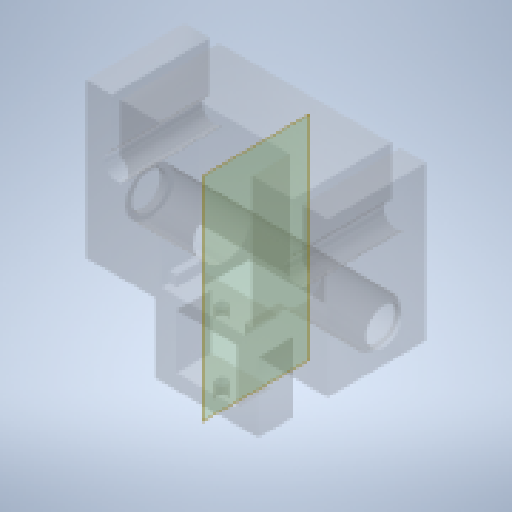
# Autodesk Inventor part: GantryHolder
Saved by Autodesk Inventor 2023 (Build 270158000, 158)
## iProperties
Created: 2022-08-28
Part Number: GantryHolder
Material: PET Plastic
Document SubType Name: Modeling
Designer: Nathann
Density: 1.541 g/cm^3
Appearance: Polycarbonate - Clear
Mass: 118.586 g
Surface Area: 221.873 cm^2
Volume: 76.9541 cm^3
Author: Nathann
Autodesk Inventor part; units mm, degrees
ref_plane "YZ Plane" through (0, 0, 0) normal (1, 0, 0) x (0, 1, 0)
ref_plane "XZ Plane" through (0, 0, 0) normal (0, 1, 0) x (-1, 0, 0)
ref_plane "XY Plane" through (0, 0, 0) normal (0, 0, 1) x (1, 0, 0)
sketch "Sketch1" plane through (0, 0, 0) normal (0, 1, 0) x (-1, 0, 0)
  arc A0 (8.5, 13.7081) -> (11.5, 13.7081) centre (10, 10) ccw
  line L0 (8.5, 20) -> (8.5, 13.7081)
  line L1 (11.5, 20) -> (11.5, 13.7081)
  line L2 (10, 20) -> (10, 18.7339)
  line L3 (20, 20) -> (10, 20)
  line L4 (8.5, 20) -> (0, 20)
  line L5 (0, 20) -> (0, 0)
  line L6 (0, 0) -> (20, 0)
  line L7 (20, 0) -> (20, 20)
  arc A1 (68.5, 13.7081) -> (71.5, 13.7081) centre (70, 10) ccw
  line L8 (68.5, 20) -> (68.5, 13.7081)
  line L9 (71.5, 20) -> (71.5, 13.7081)
  line L10 (70, 20) -> (70, 18.3732)
  line L11 (80, 20) -> (70, 20)
  line L12 (68.5, 20) -> (60.9559, 20)
  line L13 (60.9559, 20) -> (60.9559, 0)
  line L14 (60.9559, 0) -> (80, 0)
  line L15 (80, 0) -> (80, 20)
  line L16 (60.9559, 0) -> (20, 0)
  line L17 (20, 0) -> (20, 20)
  line L18 (20, 20) -> (60.9559, 20)
  line L19 (60.9559, 20) -> (60.9559, 0)
  dimension "d2" = 8
  dimension "d7" = 1.5
  dimension "d8" = 1.5
  dimension "d16" = 10
  dimension "d17" = 8
  dimension "d18" = 1.5
  dimension "d19" = 1.5
  dimension "d20" = 10
  dimension "d22" = 80
  dimension "d23" = 10
  dimension "d24" = 0
  dimension "d25" = 60
  dimension "d26" = 20
  dimension "d27" = 20
  dimension "d28" = 20
  dimension "d29" = 20
  dimension "d30" = 10
  dimension "d31" = 10
  dimension "d32" = 20
  constraints: 40 end point, 6 vertical, 5 perpendicular, 4 parallel, 4 point on circle, 3 point on line, 2 centre point, 1 horizontal
  measures "d2" diameter of A0
  measures "d7" distance between parallel lines of L0 L2
  measures "d8" distance between parallel lines of L1 L2
  measures "d16" horizontal distance of L5.end A0.centre
  measures "d17" diameter of A1
  measures "d18" distance between parallel lines of L8 L10
  measures "d19" distance between parallel lines of L9 L10
  measures "d20" vertical distance of L13.end A1.centre
  measures "d22" distance between parallel lines of L5 L15
  measures "d23" distance from line of L15 A1.centre
  measures "d24" distance between parallel lines of L6 L14
  measures "d25" distance of A0.centre A1.centre
  measures "d26" distance of L14.end L11.start
  measures "d27" distance of L12.end L13.end
  measures "d28" distance of L6.end L3.start
  measures "d29" distance of L4.end L5.end
  measures "d30" distance between parallel lines of L15 L10
  measures "d31" distance between parallel lines of L7 L2
  measures "d32" distance between parallel lines of L16 L18
extrude "Extrusion1" add sketch "Sketch1" along normal blind 36
sketch "Sketch5" plane through (-80, 0, 0) normal (-1, 0, 0) x (0, 0, 1)
  line L0 (20, 0) -> (20, 36) projected
  line L1 (20, 36) -> (-15, 36)
  line L2 (-15, 6) -> (20, 6)
  line L3 (20, 6) -> (20, 36)
  line L4 (-15, 36) -> (-15, 26.6522)
  line L5 (-15, 15.4718) -> (-15, 6)
  line L6 (0, 0) -> (0, 36) projected
  line L7 (0, 0) -> (0, 36) projected
  line L8 (0, 6) -> (0, 36)
  arc A0 (-15, 15.4718) -> (-15, 26.6522) centre (-10, 21.062) ccw
  dimension "d40" = 30
  dimension "d41" = 35
  dimension "d45" = 20
  dimension "d85" = 15
  dimension "d86" = 5
  dimension "d87" = 15
  constraints: 12 end point, 3 parallel, 2 perpendicular, 2 point on circle, 2 point on line, 1 centre point, 1 horizontal, 1 vertical
  measures "d40" distance of L1.end L2.start
  measures "d41" distance of L0.end L1.end
  measures "d45" distance between parallel lines of L0 L6
  measures "d85" diameter of A0
  measures "d86" distance from line of L4 A0.centre
  measures "d87" distance between parallel lines of L6 L5
extrude "Extrusion5" add sketch "Sketch5" against normal blind 80 contours L2 L5 A0 L4 L1 L6
sketch "Sketch13" plane through (0, 36, 0) normal (0, 1, 0) x (1, 0, 0)
  line L0 (-80, -20) -> (-80, 15) projected
  line L1 (-80, -20) -> (-71.5, -20) projected
  line L2 (-71.5, -20) -> (-71.5, -13.7081) projected
  arc A0 (-68.5, -13.7081) -> (-71.5, -13.7081) centre (-70, -10) ccw projected
  line L3 (-68.5, -13.7081) -> (-68.5, -20) projected
  line L4 (-68.5, -20) -> (-11.5, -20) projected
  line L5 (-11.5, -20) -> (-11.5, -13.7081) projected
  arc A1 (-8.5, -13.7081) -> (-11.5, -13.7081) centre (-10, -10) ccw projected
  line L6 (-8.5, -13.7081) -> (-8.5, -20) projected
  line L7 (-8.5, -20) -> (0, -20) projected
  line L8 (0, -20) -> (0, 15) projected
  line L9 (-80, 15) -> (0, 15) projected
  point P0 (0, 0)
extrude "Extrusion11" cut sketch "Sketch13" against normal blind 1
sketch "Sketch16" plane through (-80, 6, -15) normal (0, 0, -1) x (-1, 0, 0)
  line L0 (-80, -6) -> (0, -6) projected
  line L1 (0, 9.4718) -> (-80, 9.4718) projected
  line L2 (-80, -6) -> (0, -6)
  line L3 (0, -6) -> (0, 9.4718)
  line L4 (0, 9.4718) -> (-80, 9.4718)
  line L5 (-80, 9.4718) -> (-80, -6)
  line L6 (0, -6) -> (0, 29) projected
  line L7 (0, 20.6522) -> (-80, 20.6522) projected
  line L8 (0, 29) -> (-80, 29)
  line L9 (-80, 29) -> (-80, 20.6522)
  line L10 (-80, 20.6522) -> (0, 20.6522)
  line L11 (0, 20.6522) -> (0, 29)
  constraints: 16 end point, 4 parallel, 2 horizontal, 2 perpendicular
extrude "Extrusion13" add sketch "Sketch16" along normal blind 6
sketch "Sketch17" plane through (0, 0, 0) normal (0, 0, -1) x (-1, 0, 0)
  line L0 (80, 6) -> (0, 6) projected
  line L1 (0, 0) -> (80, 0) projected
  line L2 (80, 6) -> (0, 6) projected
  line L3 (80, 6) -> (80, 0)
  line L4 (0, 6) -> (0, 0)
  constraints: 4 end point, 1 parallel, 1 perpendicular
extrude "Extrusion14" add sketch "Sketch17" along normal blind 20
sketch "Sketch18" plane through (-68.5, 0, 20) normal (0, 0, 1) x (1, 0, 0)
  line L0 (13.5, 0) -> (43.5, 0)
  line L1 (43.5, 0) -> (43.5, 15)
  line L2 (43.5, 15) -> (13.5, 15)
  line L3 (13.5, 15) -> (13.5, 0)
  line L4 (-11.5, 0) -> (-11.5, 35) projected
  line L5 (0, 0) -> (57, 0) projected
  point P0 (68.5, 0)
  dimension "d128" = 15
  dimension "d129" = 8
  dimension "d130" = 8
  dimension "d148" = 0.5
  dimension "d149" = 0.5
  dimension "d107" = 30
  dimension "d108" = 25
  dimension "d109" = 15
  dimension "d110" = 0
  constraints: 8 end point, 2 parallel, 1 horizontal, 1 perpendicular
  measures "d107" distance of L1.end L2.end
  measures "d108" distance between parallel lines of L3 L4
  measures "d109" distance of L2.end L0.start
  measures "d110" distance between parallel lines of L0 L5
extrude "Extrusion15" cut sketch "Sketch18" against normal blind 37
sketch "Sketch19" plane through (0, 0, 0) normal (0, -1, 0) x (1, 0, 0)
  line L0 (-80, -21) -> (0, -21) projected
  line L1 (-30, -21) -> (-23, -21)
  line L2 (-23, -21) -> (-23, -44)
  line L3 (-23, -44) -> (-30, -44)
  line L4 (-30, -44) -> (-30, -21)
  line L5 (-30, -44) -> (-50, -44)
  line L6 (-50, -44) -> (-50, -39)
  line L7 (-50, -39) -> (-30, -39)
  line L8 (-30, -39) -> (-30, -44)
  line L9 (-50, -44) -> (-57, -44)
  line L10 (-57, -44) -> (-57, -21)
  line L11 (-57, -21) -> (-50, -21)
  line L12 (-50, -21) -> (-50, -44)
  line L13 (0, -21) -> (0, 20) projected
  point P0 (0, 0)
  dimension "d113" = 7
  dimension "d114" = 7
  dimension "d115" = 5
  dimension "d116" = 18
  dimension "d117" = 20
  dimension "d118" = 23
  constraints: 24 end point, 6 parallel, 3 horizontal, 3 perpendicular, 2 point on line
  measures "d113" distance between parallel lines of L4 L2
  measures "d114" distance between parallel lines of L10 L12
  measures "d115" distance between parallel lines of L5 L7
  measures "d116" distance between parallel lines of L0 L7
  measures "d117" distance between parallel lines of L12 L4
  measures "d118" distance between parallel lines of L13 L2
extrude "Extrusion16" add sketch "Sketch19" against normal blind 15.5 contours L0 L12 L6 L9 L10 | L0 L2 L3 L4 | L7 L4 L5 L6
sketch "Sketch20" plane through (-23, 0, -44) normal (0, 0, -1) x (-1, 0, 0)
  circle A0 centre (17, 7.5) radius 1.75
  line L0 (34, 0) -> (0, 0) projected
  line L1 (-23, 15.4718) -> (-23, 0) projected
  dimension "d121" = 3.5
  dimension "d122" = 7.5
  dimension "d123" = 40
  constraints: 1 centre point
  measures "d121" diameter of A0
  measures "d122" distance from line of L0 A0.centre
  measures "d123" distance from line of L1 A0.centre
extrude "Extrusion17" cut sketch "Sketch20" against normal blind 80
sketch "Sketch21" plane through (0, 0, 0) normal (0, -1, 0) x (1, 0, 0)
  line L0 (0, -2.5) -> (-80, -2.5) projected
  line L1 (0, -21) -> (-23, -21) projected
  line L2 (0, -21) -> (0, 20) projected
  line L3 (0, 20) -> (-8.5, 20) projected
  line L4 (-8.5, 20) -> (-8.5, 13.7081) projected
  arc A0 (-11.5, 13.7081) -> (-8.5, 13.7081) centre (-10, 10) ccw projected
  line L5 (-11.5, 13.7081) -> (-11.5, 20) projected
  line L6 (-25, 20) -> (-11.5, 20) projected
  line L7 (-25, 20) -> (-25, -17) projected
  line L8 (-25, -17) -> (-55, -17) projected
  line L9 (-55, -17) -> (-55, 20) projected
  line L10 (-68.5, 20) -> (-55, 20) projected
  line L11 (-68.5, 13.7081) -> (-68.5, 20) projected
  arc A1 (-71.5, 13.7081) -> (-68.5, 13.7081) centre (-70, 10) ccw projected
  line L12 (-71.5, 20) -> (-71.5, 13.7081) projected
  line L13 (-80, 20) -> (-71.5, 20) projected
  line L14 (-80, 20) -> (-80, -21) projected
  line L15 (-57, -21) -> (-80, -21) projected
  line L16 (-57, -21) -> (-57, -44) projected
  line L17 (-57, -44) -> (-23, -44) projected
  line L18 (-23, -44) -> (-23, -21) projected
  line L19 (-30, -21) -> (-30, -39) projected
  line L20 (-30, -39) -> (-50, -39) projected
  line L21 (-50, -39) -> (-50, -21) projected
  line L22 (-30, -21) -> (-50, -21) projected
  point P0 (0, 0)
extrude "Extrusion18" cut sketch "Sketch21" against normal blind 2.5 contours L2 L1 L18 L17 L16 L15 L14 L0 L9 L8 L7 | L0 L7 L6 L5 A0 L4 L3 L2 | L0 L14 L13 L12 A1 L11 L10 L9 | L19 L20 L21 L22
ref_plane "Work Plane5" through (-40, 21.062, -10) normal (-1, 0, 0) x (0, 0, 1)
sketch "Sketch25" plane through (-80, 6, -21) normal (0, 0, -1) x (-1, 0, 0)
  line L0 (-80, 9.4718) -> (-80, -3.5) projected
  line L1 (0, 29) -> (-80, 29) projected
  line L2 (-80, -3.5) -> (-52.5, -3.5)
  line L3 (-52.5, -3.5) -> (-52.5, 29)
  line L4 (-52.5, 29) -> (-80, 29)
  line L5 (-80, 29) -> (-80, -3.5)
  line L6 (0, 20.6522) -> (0, 29) projected
  line L7 (0, 29) -> (-27.5, 29)
  line L8 (-27.5, 29) -> (-27.5, -1)
  line L9 (-27.5, -1) -> (0, -1)
  line L10 (0, -1) -> (0, 29)
  point P0 (-80, -6)
  dimension "d138" = 27.5
  dimension "d139" = 27.5
  dimension "d140" = 30
  constraints: 16 end point, 4 parallel, 2 horizontal, 2 perpendicular, 1 point on line
  measures "d138" distance between parallel lines of L5 L3
  measures "d139" distance between parallel lines of L10 L8
  measures "d140" distance between parallel lines of L9 L1
extrude "Extrusion21" add sketch "Sketch25" against normal blind 7.5
sketch "Sketch22" plane through (-40, 21.062, -10) normal (-1, 0, 0) x (0, 0, 1)
  arc A0 (-5, -5.5902) -> (-5, 5.5902) centre (0, 0) ccw projected
  line L0 (7.5, 0) -> (-7.5, 0)
  line L1 (-7.5, 0) -> (-7.5, -8)
  line L2 (-7.5, -8) -> (7.5, -8)
  line L3 (7.5, -8) -> (7.5, 0)
  circle A1 centre (0, 0) radius 7.5
  line L4 (-7.5, 0) -> (7.5, 0)
  line L5 (7.5, 0) -> (7.5, 8)
  line L6 (7.5, 8) -> (-7.5, 8)
  line L7 (-7.5, 8) -> (-7.5, 0)
  circle A2 centre (0, 0.5) radius 7.5
  circle A3 centre (0, -0.5) radius 7.5
  point P0 (10, -21.062)
  point P1 (7.5, 0)
  point P2 (0, 0)
  point P3 (0, 0)
  point P4 (7.5, 0.5)
  point P5 (-7.5, 0.5)
  point P6 (-7.5, -0.5)
  point P7 (7.5, -0.5)
  dimension "d128" = 15
  dimension "d129" = 8
  dimension "d130" = 8
  dimension "d148" = 0.5
  dimension "d149" = 0.5
  constraints: 16 end point, 4 parallel, 3 centre point, 3 tangent, 2 horizontal, 2 midpoint, 2 perpendicular, 1 coincident, 1 concentric, 1 point on circle
  measures "d128" distance between parallel lines of L3 L1
  measures "d129" distance between parallel lines of L2 L0
  measures "d130" distance between parallel lines of L0 L6
  measures "d148" distance of point (0, 0) A2.centre
  measures "d149" distance of point (0, 0) A3.centre
extrude "Extrusion19" cut sketch "Sketch22" along normal mid plane 75 contours A1 A3 A2 A0 | A0 A3 A1 | A3 L0 A0 | A0 L3 A3 | A3 L1 A1 | A1 L0 A3 | L0 A2 A0 | A0 A2 L5 | A2 L0 | A3 A2 A1 A0 | L0 A3 | A1 A2 L0 | L7 A2 A1 | A0 A1 A2
sketch "Sketch24" plane through (-80, 6, -21) normal (0, 0, -1) x (-1, 0, 0)
  line L0 (0, 29) -> (-80, 29) projected
  line L1 (-27.5, 29) -> (-52.5, 29)
  line L2 (-52.5, 29) -> (-52.5, 8.062)
  line L3 (-52.5, 8.062) -> (-27.5, 8.062)
  line L4 (-27.5, 8.062) -> (-27.5, 29)
  line L5 (0, 20.6522) -> (0, 29) projected
  line L6 (-80, 9.4718) -> (-80, -3.5) projected
  line L7 (-52.5, 29) -> (-80, 29)
  line L8 (-80, 29) -> (-80, -3.5)
  line L9 (-80, -3.5) -> (-52.5, -3.5)
  line L10 (-52.5, -3.5) -> (-52.5, 29)
  line L11 (0, -3.5) -> (0, 9.4718) projected
  line L12 (-27.5, 29) -> (0, 29)
  line L13 (0, 29) -> (0, -3.5)
  line L14 (0, -3.5) -> (-27.5, -3.5)
  line L15 (-27.5, -3.5) -> (-27.5, 29)
  line L16 (-77.5, 23.062) -> (-2.5, 23.062) projected
  line L17 (-27.5, 23.062) -> (-52.5, 23.062)
  line L18 (-52.5, 23.062) -> (-52.5, 1.5824)
  line L19 (-52.5, 1.5824) -> (-27.5, 1.5824)
  line L20 (-27.5, 1.5824) -> (-27.5, 23.062)
  point P0 (-80, -6)
  point P1 (-27.5, 23.062)
  dimension "d133" = 25
  dimension "d134" = 27.5
  dimension "d135" = 15
  constraints: 32 end point, 8 parallel, 4 horizontal, 4 perpendicular, 4 point on line
  measures "d133" distance between parallel lines of L2 L4
  measures "d134" distance between parallel lines of L5 L4
  measures "d135" distance between parallel lines of L3 L16
extrude "Extrusion20" cut sketch "Sketch24" against normal blind 10 contours L4 L3 L2 L16
sketch "Sketch26" plane through (0, 35, 20) normal (1, 0, 0) x (0, 0, -1)
  arc A0 (33.5, -7.3047) -> (33.5, -20.5712) centre (30, -13.938) ccw projected
  circle A1 centre (30, -13.938) radius 6
  line L0 (41, 0) -> (41, -32.5) projected
  line L1 (0, 0) -> (41, 0) projected
  line L2 (0, -32.5) -> (0, 0) projected
  line L3 (0, -32.5) -> (41, -32.5) projected
  line L4 (33.5, -20.5712) -> (33.5, -7.3047) projected
  arc A2 (33.5, -7.3047) -> (33.5, -20.5712) centre (30, -13.938) ccw projected
  point P0 (20, -35)
  point P1 (35, -8.3478)
  point P2 (35, -19.5282)
  dimension "d143" = 12
  constraints: 1 centre point, 1 coincident
  measures "d143" diameter of A1
extrude "Extrusion22" add sketch "Sketch26" against normal blind 2.5 contours L4 A1 A0
sketch "Sketch27" plane through (-80, 35, -21) normal (-1, 0, 0) x (0, 0, 1)
  arc A0 (7.5, -20.5712) -> (7.5, -7.3047) centre (11, -13.938) ccw projected
  line L0 (7.5, -7.3047) -> (7.5, -20.5712) projected
  line L1 (0, -32.5) -> (0, 0) projected
  line L2 (0, -32.5) -> (41, -32.5) projected
  line L3 (41, -32.5) -> (41, 0) projected
  line L4 (41, 0) -> (0, 0) projected
  circle A1 centre (11, -13.938) radius 6
  point P0 (21, -35)
  constraints: 1 centre point, 1 coincident
extrude "Extrusion23" add sketch "Sketch27" against normal blind 2.5 contours L0 A1 A0
sketch "Sketch28" plane through (-80, 6, -21) normal (0, 0, -1) x (-1, 0, 0)
  line L0 (-77.5, 23.062) -> (-2.5, 23.062) projected
  line L1 (-57.32, 23.062) -> (-20.6249, 23.062)
  line L2 (-20.6249, 23.062) -> (-20.6249, 8)
  line L3 (-20.6249, 8) -> (-57.32, 8)
  line L4 (-57.32, 8) -> (-57.32, 23.062)
  line L5 (-57, 9.5) -> (-23, 9.5) projected
  point P0 (-80, -6)
  dimension "d152" = 1.5
  constraints: 8 end point, 2 parallel, 1 horizontal, 1 perpendicular, 1 point on line
  measures "d152" distance between parallel lines of L3 L5
extrude "Extrusion24" cut sketch "Sketch28" along normal blind 30.5
sketch "Sketch29" plane through (-80, 35, -21) normal (-1, 0, 0) x (0, 0, 1)
  arc A0 (7.5, -18.8114) -> (7.5, -9.0646) centre (11, -13.938) ccw projected
  circle A1 centre (11, -13.938) radius 6
  point P0 (21, -35)
  point P1 (7.5, -9.0646)
  point P2 (7.5, -18.8114)
  constraints: 1 centre point, 1 coincident
extrude "Extrusion25" cut sketch "Sketch29" against normal blind 100.5
sketch "Sketch30" plane through (-68.5, 35, 20) normal (0, 0, 1) x (1, 0, 0)
  line L0 (-11.5, -32.5) -> (-3, -32.5) projected
  line L1 (-3, -32.5) -> (-3, 0) projected
  line L2 (-3, 0) -> (-11.5, 0) projected
  line L3 (-11.5, -32.5) -> (-11.5, 0) projected
  line L4 (0, -32.5) -> (13.5, -32.5) projected
  line L5 (13.5, -32.5) -> (13.5, -20) projected
  line L6 (13.5, -20) -> (43.5, -20) projected
  line L7 (43.5, -20) -> (43.5, -32.5) projected
  line L8 (43.5, -32.5) -> (57, -32.5) projected
  line L9 (57, -32.5) -> (57, 0) projected
  line L10 (57, 0) -> (0, 0) projected
  line L11 (0, -32.5) -> (0, 0) projected
  line L12 (60, -32.5) -> (68.5, -32.5) projected
  line L13 (68.5, -32.5) -> (68.5, 0) projected
  line L14 (68.5, 0) -> (60, 0) projected
  line L15 (60, -32.5) -> (60, 0) projected
  point P0 (68.5, -35)
extrude "Extrusion26" add sketch "Sketch30" along normal blind 15
sketch "Sketch31" plane through (-68.5, 35, 35) normal (0, 0, 1) x (1, 0, 0)
  line L0 (-11.5, 0) -> (68.5, 0) projected
  line L1 (43.5, -32.5) -> (57, -32.5) projected
  line L2 (8.5, 0) -> (50.25, 0)
  line L3 (50.25, 0) -> (50.25, -32.5)
  line L4 (50.25, -32.5) -> (8.5, -32.5)
  line L5 (8.5, -32.5) -> (8.5, 0)
  line L6 (-11.5, 0) -> (-11.5, -32.5) projected
  line L7 (48.5, -32.5) -> (48.5, 0)
  line L8 (68.5, -32.5) -> (68.5, 0) projected
  point P0 (68.5, -35)
  dimension "d157" = 20
  dimension "d158" = 20
  constraints: 10 end point, 3 point on line, 2 parallel, 2 perpendicular, 1 horizontal, 1 midpoint
  measures "d157" distance between parallel lines of L6 L5
  measures "d158" distance between parallel lines of L8 L7
extrude "Extrusion27" cut sketch "Sketch31" against normal blind 15 contours L0 L7 L1 L4 L5
equation "\"d2\" = RodDiameter"
equation "\"d17\" = d2"
equation "\"d130\" = d129"
equation "\"d139\" = d138"
equation "\"RodDiameter\" = 8"
equation "\"VerticalBearingOD\" = 16"
equation "\"PrintingClearance\" = 0.2"
equation "\"d21\" = 8"
equation "\"TubeID\" = 18"
body "Solid1"
